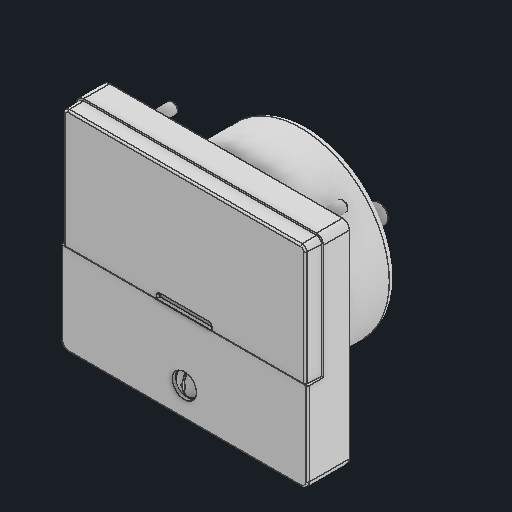
# Autodesk Inventor part: BaomainPanelMountMeter
Saved by Autodesk Inventor 2025.2 (Build 292293000, 293)
## iProperties
Created: 2025-09-23
Part Number: BaomainPanelMountMeter
Material: Generic
Document SubType Name: Modeling
Designer: valer
Density: 1 g/cm^3
Appearance: Default
Author: valer
Autodesk Inventor part; units mm, degrees
ref_plane "YZ Plane" through (0, 0, 0) normal (1, 0, 0) x (0, 1, 0)
ref_plane "XZ Plane" through (0, 0, 0) normal (0, 1, 0) x (-1, 0, 0)
ref_plane "XY Plane" through (0, 0, 0) normal (0, 0, 1) x (1, 0, 0)
sketch "Base" plane through (0, 0, 0) normal (0, 0, 1) x (1, 0, 0)
  line L0 (-35.5, -30.5) -> (35.5, -30.5)
  line L1 (35.5, -30.5) -> (35.5, 30.5)
  line L2 (35.5, 30.5) -> (-35.5, 30.5)
  line L3 (-35.5, 30.5) -> (-35.5, -30.5)
  line L4 (-35.5, -30.5) -> (35.5, 30.5) construction
  line L5 (35.5, -30.5) -> (-35.5, 30.5) construction
  point P0 (0, 0)
  dimension "d0" = 71
  dimension "d1" = 61
  constraints: 12 end point, 2 midpoint, 2 parallel, 1 horizontal, 1 perpendicular
  measures "d0" distance of L1.end L2.end
  measures "d1" distance of L2.end L0.start
extrude "BaseFeature" add sketch "Base" along normal blind 12
sketch "Sketch2" plane through (0, 0, 12) normal (0, 0, 1) x (1, 0, 0)
  line L0 (35.5, 30.5) -> (-35.5, 30.5) projected
  line L1 (-35.5, 30.5) -> (35.5, 30.5)
  line L2 (35.5, 30.5) -> (35.5, -4.5)
  line L3 (35.5, -4.5) -> (-35.5, -4.5)
  line L4 (-35.5, -4.5) -> (-35.5, 30.5)
  point P0 (0, 0)
  dimension "d4" = 35
  constraints: 8 end point, 2 parallel, 1 horizontal, 1 perpendicular
  measures "d4" distance between parallel lines of L0 L3
extrude "Extrusion2" cut sketch "Sketch2" against normal blind 4.5
fillet "Fillet1" radius 2 4 edges at (35.5, -30.5, 6) (-35.5, -30.5, 6) (35.5, 30.5, 3.75) (-35.5, 30.5, 3.75)
fillet "Fillet2" radius 0.5 5 edges at (-34.9142, -29.9142, 12) (0, -30.5, 12) (34.9142, -29.9142, 12) (35.5, -16.5, 12) (-35.5, -16.5, 12)
sketch "Sketch3" plane through (0, 0, 12) normal (0, 0, 1) x (1, 0, 0)
  line L0 (0, -30.5) -> (0, -4.5) construction
  line L1 (35, -4.5) -> (-35, -4.5) projected
  line L2 (0, -57.249) -> (0, 45.1248) construction
  line L3 (-33.5, -30.5) -> (33.5, -30.5) construction
  circle A0 centre (0, -22) radius 3.5
  point P0 (0, 0)
  dimension "d9" = 7
  dimension "d10" = 8.5
  constraints: 2 end point, 2 midpoint, 1 centre point, 1 collinear, 1 point on line
  measures "d9" diameter of A0
  measures "d10" distance from line of L3 A0.centre
extrude "Extrusion3" cut sketch "Sketch3" against normal blind 1
sketch "Sketch4" plane through (0, -22, 11) normal (0, 0, 1) x (1, 0, 0)
  circle A0 centre (0, 0) radius 3.5 projected
  circle A1 centre (0, 0) radius 3.25
  point P0 (0, 22)
  dimension "d13" = 0.25
  constraints: 1 centre point, 1 coincident
  measures "d13" radial gap between concentric circles of A0 A1
extrude "Extrusion4" add sketch "Sketch4" along normal blind 1.25 contours A1
fillet "Fillet3" radius 3.2 1 edges at (-3.25, -22, 12.25)
sketch "Sketch5" plane through (0, -22, 12.25) normal (0, 0, 1) x (1, 0, 0)
  line L0 (0, 3.25) -> (0, -3.25) construction
  circle A0 centre (0, 0) radius 3.25 projected
  line L1 (-0.25, -3) -> (0.25, -3)
  line L2 (0.25, -3) -> (0.25, 3)
  line L3 (0.25, 3) -> (-0.25, 3)
  line L4 (-0.25, 3) -> (-0.25, -3)
  line L5 (-0.25, -3) -> (0.25, 3) construction
  line L6 (0.25, -3) -> (-0.25, 3) construction
  point P0 (0, 22)
  dimension "d17" = 0.5
  dimension "d18" = 6
  constraints: 14 end point, 3 midpoint, 2 parallel, 2 point on circle, 1 horizontal, 1 perpendicular, 1 vertical
  measures "d17" distance of L2.end L3.end
  measures "d18" distance of L1.end L2.end
extrude "Extrusion5" cut sketch "Sketch5" against normal blind 1 contours L4 L3 L2 L1
sketch "Sketch6" plane through (0, 0, 7.5) normal (0, 0, 1) x (1, 0, 0)
  line L0 (-35.5, -4.5) -> (-35.5, 28.5) projected
  arc A0 (-33.5, 30.5) -> (-35.5, 28.5) centre (-33.5, 28.5) ccw projected
  line L1 (-33.5, 30.5) -> (33.5, 30.5) projected
  arc A1 (35.5, 28.5) -> (33.5, 30.5) centre (33.5, 28.5) ccw projected
  line L2 (35.5, 28.5) -> (35.5, -4.5) projected
  line L3 (35, -4.5) -> (35, 28.5)
  arc A2 (35, 28.5) -> (33.5, 30) centre (33.5, 28.5) ccw
  line L4 (33.5, 30) -> (-33.5, 30)
  arc A3 (-33.5, 30) -> (-35, 28.5) centre (-33.5, 28.5) ccw
  line L5 (-35, 28.5) -> (-35, -4.5)
  line L6 (-35, -4.5) -> (35, -4.5)
  line L7 (35.5, -4.5) -> (-35.5, -4.5) projected
  point P0 (0, 0)
  dimension "d21" = 0.5
  constraints: 8 end point, 4 point on circle, 2 centre point, 1 collinear, 4 other
  measures "d21" distance between parallel lines of L1 L4
extrude "Extrusion6" add sketch "Sketch6" along normal up to surface (4.5 mm away) draft -2 contours L5 A3 L4 A2 L3 L6
fillet "Fillet4" radius 0.5 5 edges at (-34.4495, 29.4495, 12) (0, 29.8429, 12) (34.4495, 29.4495, 12) (34.8429, 12.0786, 12) (-34.8429, 12.0786, 12)
sketch "Sketch7" plane through (-34.36, -4.3429, 12) normal (0, 0, 1) x (1, 0, 0)
  circle A0 centre (34.36, -17.6571) radius 3.5 projected
  line L0 (0.86, 33.7029) -> (67.86, 33.7029) projected
  line L1 (34.36, -17.6571) -> (31.914, -15.1538)
  line L2 (68.72, 0) -> (0, 0) projected
  line L3 (26.36, 0) -> (42.36, 0)
  line L4 (42.36, 0) -> (42.36, 1.9016)
  line L5 (42.36, 1.9016) -> (26.36, 1.9016)
  line L6 (26.36, 1.9016) -> (26.36, 0)
  line L7 (34.36, 1.9016) -> (34.36, -17.6571)
  point P0 (42.36, 0)
  dimension "d28" = 16
  constraints: 12 end point, 2 parallel, 2 perpendicular, 1 coincident, 1 horizontal, 1 midpoint, 1 point on line, 2 other
  measures "d28" distance of L4.end L5.end
extrude "Extrusion7" cut sketch "Sketch7" against normal blind 1 contours L2 L7 L5 L4 | L2 L6 L5 L7
fillet "Fillet5" radius 1 2 edges at (-8, -2.4412, 11.5) (8, -2.4412, 11.5)
sketch "Sketch8" plane through (0, 0, 0) normal (0, 0, -1) x (-1, 0, 0)
  circle A0 centre (0, 0) radius 25.5
  dimension "d32" = 51
  constraints: 1 centre point, 1 coincident
  measures "d32" diameter of A0
extrude "Extrusion8" add sketch "Sketch8" along normal blind 23.5
fillet "Fillet6" radius 2 1 edges at (25.5, 0, -23.5)
sketch "Sketch9" plane through (0, 0, -23.5) normal (0, 0, -1) x (-1, 0, 0)
  line L0 (0, 0) -> (0, -25.5) construction
  circle A0 centre (0, -22) radius 3.5 construction
  circle A1 centre (0, -12.75) radius 10.75
  constraints: 2 end point, 1 centre point, 1 midpoint, 1 vertical, 1 vertical alignment, 1 other
extrude "Extrusion9" add sketch "Sketch9" along normal blind 5.5
fillet "Fillet7" radius 2 1 edges at (10.75, -12.75, -29)
sketch "Sketch10" plane through (0, 0, -23.5) normal (0, 0, -1) x (-1, 0, 0)
  line L0 (-14.5, 7.5) -> (14.5, 7.5) construction
  line L1 (0, 0) -> (0, 23.5) construction
  circle A0 centre (0, 0) radius 23.5 projected
  circle A1 centre (-14.5, 7.5) radius 2.665
  circle A2 centre (14.5, 7.5) radius 2.665
  line L2 (-33.5, 30.5) -> (33.5, 30.5) projected
  point P0 (0, -23.5)
  point P1 (0, 7.5)
  dimension "d39" = 5.33
  dimension "d40" = 29
  dimension "d41" = 23
  constraints: 4 end point, 2 centre point, 2 coincident, 1 equal radius, 1 horizontal, 1 midpoint, 1 point on circle, 1 point on line, 1 vertical
  measures "d39" diameter of A1
  measures "d40" distance of L0.start L0.end
  measures "d41" distance between parallel lines of L2 L0
extrude "Extrusion10" add sketch "Sketch10" along normal blind 6 contours A1 | A2
sketch "Sketch11" plane through (0, 0, 0) normal (0, 0, -1) x (-1, 0, 0)
  circle A0 centre (-24.5, -24.5) radius 1.5
  circle A1 centre (24.5, -24.5) radius 1.5
  line L0 (49.7, 0) -> (-49.7, 0) construction
  line L1 (-24.5, -24.5) -> (24.5, -24.5) construction
  line L2 (0, -42.7) -> (0, 42.7) construction
  circle A2 centre (-24.5, 24.5) radius 1.5
  circle A3 centre (24.5, 24.5) radius 1.5
  line L3 (-24.5, 24.5) -> (24.5, 24.5) construction
  point P0 (0, 0)
  point P1 (0, -24.5)
  dimension "d44" = 3
  dimension "d45" = 49
  dimension "d46" = 49
  constraints: 4 centre point, 4 end point, 2 symmetric about line, 1 equal radius, 1 horizontal, 1 midpoint, 1 point on line, 2 other
  measures "d44" diameter of A1
  measures "d45" distance of L1.start L1.end
  measures "d46" distance between parallel lines of L1 L3
extrude "Extrusion11" add sketch "Sketch11" along normal blind 9.5
chamfer "Chamfer1" distance 0.5 angle 45 4 edges at (26, 24.5, -9.5) (26, -24.5, -9.5) (-23, -24.5, -9.5) (-23, 24.5, -9.5)
body "Solid1"
